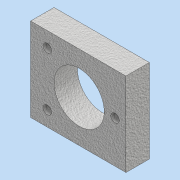
# Autodesk Inventor part: Uchwyt górnego łożyska osi Z
Saved by Autodesk Inventor 2018 (Build 220112000, 112)
## iProperties
Created: 2019-02-03
Part Number: Uchwyt górnego łożyska osi Z
Material: Ogólny
Document SubType Name: Modeling
Designer: Dawid
Density: 1 g/cm^3
Appearance: Aluminium odlewane
Author: Dawid
Autodesk Inventor part; units mm, degrees
ref_plane "YZ Plane" through (0, 0, 0) normal (1, 0, 0) x (0, 1, 0)
ref_plane "XZ Plane" through (0, 0, 0) normal (0, 1, 0) x (-1, 0, 0)
ref_plane "XY Plane" through (0, 0, 0) normal (0, 0, 1) x (1, 0, 0)
sketch "Szkic1" plane through (0, 0, 0) normal (0, 1, 0) x (-1, 0, 0)
  circle A0 centre (3, 0) radius 15
  line L0 (32, -51.5) -> (19.7697, -51.5)
  arc A1 (19.7697, -48.5) -> (19.7697, -51.5) centre (15, -50) ccw
  line L1 (19.7697, -48.5) -> (32, -48.5)
  line L2 (32, 48.5) -> (32, -48.5)
  line L3 (32, 48.5) -> (19.7697, 48.5)
  arc A2 (19.7697, 51.5) -> (19.7697, 48.5) centre (15, 50) ccw
  line L4 (19.7697, 51.5) -> (32, 51.5)
  line L5 (32, 60) -> (32, 51.5)
  line L6 (32, 60) -> (-25, 60)
  line L7 (-25, 60) -> (-25, -60)
  line L8 (-25, -60) -> (32, -60)
  line L9 (32, -51.5) -> (32, -60)
  line L10 (-25, 0) -> (-25, -25)
  line L11 (-25, -25) -> (32, -25)
  line L12 (-25, 0) -> (-25, 25)
  line L13 (-25, 25) -> (32, 25)
  point P0 (0, 0)
  point P1 (0, 0)
  dimension "d0" = 25
  dimension "d1" = 25
  constraints: 28 end point, 4 point on circle, 4 point on line, 3 centre point, 2 perpendicular, 1 midpoint
  measures "d0" distance of L10.start L10.end
  measures "d1" distance of L10.start L12.end
extrude "Wyciągnięcie proste1" add sketch "Szkic1" along normal blind 14 contours L7 L13 L2 L11
sketch "Szkic2" plane through (0, 14, 0) normal (0, 1, 0) x (1, 0, 0)
  circle A0 centre (-3, 0) radius 15 projected
  line L0 (-32, 25) -> (-32, -25) projected
  line L1 (25, -25) -> (25, 25) projected
  line L2 (12, 0) -> (15, 0)
  line L3 (-18, 0) -> (-22, 0)
  line L4 (-22, 0) -> (-22, 16)
  line L5 (-22, 0) -> (-22, -16)
  circle A1 centre (-22, 16) radius 2.5
  circle A2 centre (-22, -16) radius 2.5
  line L6 (12, 0) -> (18.5, 0)
  circle A3 centre (18.5, 0) radius 2.5
  point P0 (0, 0)
  dimension "d11" = 10
  dimension "d12" = 5
  dimension "d13" = 5
  dimension "d18" = 6.5
  dimension "d19" = 5
  constraints: 10 end point, 3 centre point, 3 coincident, 3 horizontal, 2 point on circle, 1 perpendicular, 1 vertical
  measures "d11" distance between parallel lines of L0 L4
  measures "d12" diameter of A1
  measures "d13" diameter of A2
  measures "d18" distance of L2.start L6.end
  measures "d19" diameter of A3
extrude "Wyciągnięcie proste2" cut sketch "Szkic2" against normal up to next contours A2 | A1 | A3
